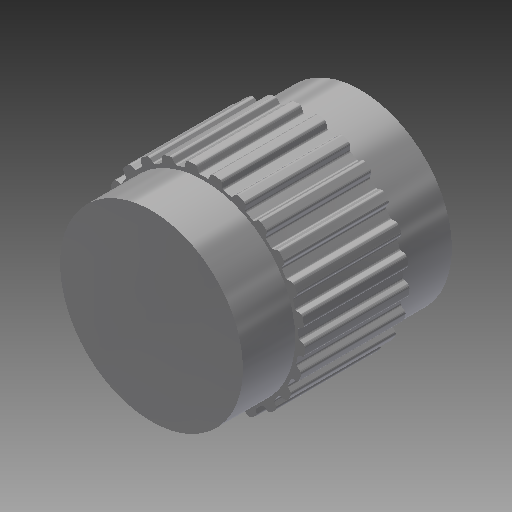
# Autodesk Inventor part: Synchronous Pulley2
Saved by Autodesk Inventor 2018 (Build 220112000, 112)
## iProperties
Created: 2020-03-19
Part Number: Synchronous Pulley2
Material: Steel
Document SubType Name: Modeling
Designer: Bunny320
Density: 1 g/cm^3
Appearance: Steel
CustomPartVersion: 1
Author: Bunny320
Autodesk Inventor part; units mm, degrees
ref_plane "YZ Plane" through (0, 0, 0) normal (1, 0, 0) x (0, 1, 0)
ref_plane "XZ Plane" through (0, 0, 0) normal (0, 1, 0) x (-1, 0, 0)
ref_plane "XY Plane" through (0, 0, 0) normal (0, 0, 1) x (1, 0, 0)
sketch "Pulley Sketch" plane through (0, 0, 0) normal (0, 0, 1) x (1, 0, 0)
  circle A0 centre (0, 0) radius 19.8944 construction
  circle A1 centre (0, 0) radius 19.3944
  circle A2 centre (0, 0) radius 18.1444
  line L0 (-1.4573, 19.3395) -> (-0.9, 18.1444)
  line L1 (-0.9, 18.1444) -> (0.9, 18.1444)
  line L2 (0.9, 18.1444) -> (1.4573, 19.3395)
  line L3 (0, 0) -> (0, 19.3944) construction
  point P0 (0, 18.1444)
  dimension "d0" = 39.7887
  dimension "d1" = 0.5
  dimension "d2" = 1.25
  dimension "d3" = 50
  dimension "d4" = 1.8
  constraints: 8 end point, 3 coincident, 3 point on circle, 2 centre point, 1 horizontal, 1 midpoint, 1 point on line, 1 vertical, 1 vertical alignment, 3 other
  measures "d0" diameter of A0
  measures "d1" radial gap between concentric circles of A0 A1
  measures "d3" angle of L2 L0
  measures "d4" distance of L0.end L1.end
extrude "Base Body" add sketch "Pulley Sketch" along normal mid plane 20 contours A2 | A1 L0 L1 L2 | L2 L1 L0 A1
extrude "Tooth" cut sketch "Pulley Sketch" along normal through all both and the other way through all contours L2 L1 L0 A1 picked at (0, 18.9737)
fillet "Tooth Fillet" radius 0.4 2 edges at (0.9, 18.1444, 0) (-0.9, 18.1444, 0)
fillet "Tooth Fillet" radius 0.6 4 edges at (-1.4573, 19.3395, 5) (-1.4573, 19.3395, -5) (1.4573, 19.3395, 5) (1.4573, 19.3395, -5)
pattern_circular "Teeth" count 25 over 360 about axis through (0, 0, -10) along (0, 0, 1) of "Tooth", "Tooth Fillet"
feature "Left flange" [suppressed]
feature "Right flange" [suppressed]
sketch "Sketch2" plane through (0, 0, 0) normal (0, 0, 1) x (1, 0, 0)
  circle A0 centre (0, 0) radius 17.5
  dimension "d17" = 35
  constraints: 1 centre point, 1 coincident
  measures "d17" diameter of A0
extrude "Extrusion3" add sketch "Sketch2" along normal mid plane 40
equation "\"d1\" = da_a"
equation "\"d2\" = da_hg"
equation "\"d3\" = 2 * da_fi"
equation "\"d4\" = da_bw"
equation "\"d5\" = da_bf"
equation "\"d7\" = da_bf"
equation "\"d9\" = da_rb"
equation "\"d10\" = da_rt"
equation "\"da_pb\" = 5"
equation "\"da_fi\" = 25deg"
equation "\"da_hg\" = 1.25"
equation "\"da_bw\" = 1.8"
equation "\"da_rb\" = 0.4"
equation "\"da_rt\" = 0.6"
equation "\"da_a\" = 0.5"
equation "\"da_bf\" = 20"
equation "\"da_wf\" = 1"
equation "\"da_hf\" = 1.2"
body "Solid1"
